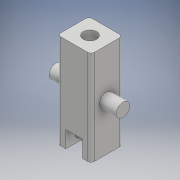
# Autodesk Inventor part: Ante pierna
Saved by Autodesk Inventor 2017 (Build 210142000, 142)
## iProperties
Part Number: Ante pierna
Material: Genérico
Document SubType Name: Modeling
Designer: HOME
Density: 1 g/cm^3
Appearance: Valor por defecto
Author: HOME
Autodesk Inventor part; units mm, degrees
ref_plane "YZ Plane" through (0, 0, 0) normal (1, 0, 0) x (0, 1, 0)
ref_plane "XZ Plane" through (0, 0, 0) normal (0, 1, 0) x (-1, 0, 0)
sketch "Boceto1" plane through (0, 0, 0) normal (0, 0, 1) x (1, 0, 0)
  line L0 (0, 0) -> (20, 0)
  line L1 (20, 0) -> (20, 18.75)
  line L2 (20, 18.75) -> (0, 18.75)
  line L3 (0, 18.75) -> (0, 0)
  point P0 (9.375, 9.375)
  dimension "d0" = 20
  dimension "d10" = 18.75
  constraints: 8 end point, 3 perpendicular, 1 vertical, 1 other
  measures "d0" distance of L0.start L0.end
  measures "d10" distance of L0.end L1.end
extrude "Extrusión1" add sketch "Boceto1" against normal blind 56.25
sketch "Boceto2" plane through (0, 0, 0) normal (0, 0, 1) x (1, 0, 0)
  circle A0 centre (10, 9.375) radius 4
  line L0 (0, 0) -> (20, 0) projected
  line L1 (0, 18.75) -> (0, 0) projected
  point P0 (10, 0)
  point P1 (0, 9.375)
  dimension "d3" = 8
  constraints: 2 midpoint, 1 centre point, 1 horizontal alignment, 1 vertical alignment
  measures "d3" diameter of A0
extrude "Extrusión2" cut sketch "Boceto2" against normal blind 10
fillet "Empalme1" radius 2 4 edges at (20, 0, -28.125) (0, 0, -28.125) (0, 18.75, -28.125) (20, 18.75, -28.125)
sketch "Boceto3" plane through (0, 0, -56.25) normal (0, 0, -1) x (-1, 0, 0)
  line L0 (-20, 16.75) -> (-20, 2) projected
  line L1 (-18, 0) -> (-2, 0) projected
  line L2 (-5, 18.75) -> (-15, 18.75)
  line L3 (-15, 18.75) -> (-15, 0)
  line L4 (-15, 0) -> (-5, 0)
  line L5 (-5, 0) -> (-5, 18.75)
  line L6 (-5, 18.75) -> (-15, 0) construction
  line L7 (-15, 18.75) -> (-5, 0) construction
  line L8 (-2, 18.75) -> (-18, 18.75) projected
  point P0 (0, 0)
  point P1 (-10, 10)
  point P2 (-10, 9.375)
  dimension "d11" = 10
  constraints: 12 end point, 3 perpendicular, 2 midpoint, 1 parallel, 1 point on line
  measures "d11" distance of L2.start L2.end
extrude "Extrusión3" cut sketch "Boceto3" against normal blind 10
ref_plane "Plano de trabajo4" through (10, 0, 0) normal (1, 0, 0) x (0, 1, 0)
sketch "Boceto5" plane through (0, 2, 0) normal (-1, 0, 0) x (0, 0, 1)
  circle A0 centre (-28.125, 7) radius 4
  line L0 (0, 14.75) -> (0, 0) projected
  line L1 (0, 0) -> (-56.25, 0) projected
  point P0 (0, -2)
  dimension "d20" = 8
  dimension "d21" = 28.125
  dimension "d22" = 7
  constraints: 1 centre point
  measures "d20" diameter of A0
  measures "d21" distance from line of A0.centre L0
  measures "d22" distance from line of A0.centre L1
extrude "Extrusión5" add sketch "Boceto5" along normal blind 10 and the other way blind 30
sketch "Boceto6" plane through (15, 0, -56.25) normal (-1, 0, 0) x (0, 0, 1)
  line L0 (0, 0) -> (56.25, 0) projected
  line L1 (56.25, 13.375) -> (56.25, 5.375) projected
  arc A0 (2.5, 12.4975) -> (7.5, 12.4975) centre (5, 9.375) ccw
  line L2 (2.5, 12.4975) -> (7.5, 12.4975)
  line L3 (7.5, 12.4975) -> (7.5, 7.9975)
  line L4 (7.5, 7.9975) -> (2.5, 7.9975)
  line L5 (2.5, 7.9975) -> (2.5, 12.4975)
  dimension "d38" = 8
  dimension "d39" = 9.375
  dimension "d40" = 51.25
  dimension "d41" = 5
  dimension "d42" = 4.5
  constraints: 8 end point, 2 horizontal, 2 point on circle, 1 centre point, 1 parallel, 1 vertical
  measures "d38" diameter of A0
  measures "d39" distance from line of L0 A0.centre
  measures "d40" distance from line of L1 A0.centre
  measures "d41" distance of L2.start L2.end
  measures "d42" distance of L4.end L2.start
extrude "Extrusión6" add sketch "Boceto6" along normal up to next contours L5 L4 L3 A0
